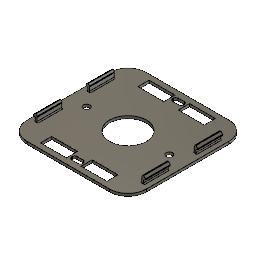
LightSwitch (Autodesk Fusion 360 design; units mm, degrees)
Autodesk Fusion 360 part; units mm, degrees
sketch "Sketch1" plane through (0, 0, 0) normal (0, 1, 0) x (1, 0, 0)
  line L0 (32.5, 32.5) -> (-32.5, -32.5) construction
  line L1 (-32.5, 32.5) -> (32.5, -32.5) construction
  line L2 (25.4289, -32.5) -> (32.5, -25.4289)
  line L3 (32.5, 25.4289) -> (25.4289, 32.5)
  line L4 (-25.4289, 32.5) -> (-32.5, 25.4289)
  line L5 (-32.5, -25.4289) -> (-25.4289, -32.5)
  line L6 (-32.5, 32.5) -> (-32.5, 25.4289)
  line L7 (-32.5, -25.4289) -> (-32.5, -32.5)
  line L8 (-32.5, 25.4289) -> (-32.5, -25.4289)
  line L9 (32.5, 32.5) -> (25.4289, 32.5)
  line L10 (-25.4289, 32.5) -> (-32.5, 32.5)
  line L11 (25.4289, 32.5) -> (-25.4289, 32.5)
  line L12 (-32.5, -32.5) -> (-25.4289, -32.5)
  line L13 (25.4289, -32.5) -> (32.5, -32.5)
  line L14 (-25.4289, -32.5) -> (25.4289, -32.5)
  line L15 (32.5, -32.5) -> (32.5, -25.4289)
  line L16 (32.5, 25.4289) -> (32.5, 32.5)
  line L17 (32.5, -25.4289) -> (32.5, 25.4289)
  line L18 (24.7919, 30.962) -> (-24.7919, 30.962)
  line L19 (-24.7919, 30.962) -> (-30.962, 24.7919)
  line L20 (-30.962, 24.7919) -> (-30.962, -24.7919)
  line L21 (-30.962, -24.7919) -> (-24.7919, -30.962)
  line L22 (-24.7919, -30.962) -> (24.7919, -30.962)
  line L23 (24.7919, -30.962) -> (30.962, -24.7919)
  line L24 (30.962, -24.7919) -> (30.962, 24.7919)
  line L25 (30.962, 24.7919) -> (24.7919, 30.962)
  dimension "d1" = 65
  dimension "d2" = 65
  dimension "d3" = 10
  dimension "d6" = 360
  dimension "d10" = 7.0711
  dimension "d11" = 1.538
extrude "Extrude1" add sketch "Sketch1" along normal blind 1.5 contours L2 L3 L4 L5 L8 L11 L14 L17 | L2 L13 L15 | L5 L7 L12 | L3 L9 L16 | L4 L6 L10 | L18 L19 L20 L21 L22 L23 L24 L25 makes body 1
extrude "Extrude2" add 1 faces at (8.4763, 1.5, 10.8333) along direction (0, 1, 0) blind 10 on bodies 1 bodies 1
delete_face "DeleteFace1" 1 faces at (-32.5, 3.8333, 27.786) on bodies 1
delete_face "DeleteFace2" 1 faces at (27.786, 7.6667, 32.5) on bodies 1
delete_face "DeleteFace3" 1 faces at (32.5, 3.8333, -27.786) on bodies 1
delete_face "DeleteFace4" 1 faces at (-27.786, 3.8333, -32.5) on bodies 1
fillet "Fillet1" radius 5 4 edges at (0, 11.5, 32.5) (-32.5, 11.5, 0) (0, 11.5, -32.5) (32.5, 11.5, 0) on bodies 1
fillet "Fillet1" radius 10 4 edges at (-32.5, 5.75, -32.5) (-32.5, 5.75, 32.5) (32.5, 5.75, 32.5) (32.5, 5.75, -32.5) on bodies 1
shell "Shell1" thickness 1.5 removed faces 0 bodies 1
ref_plane "WorkPlane1" through (28.9645, 1.5, -28.9645) normal (0, 1, 0) x (1, 0, 0)
split "Split1" by plane through (28.9645, 1.5, -28.9645) normal (0, 1, 0) bodies 1 makes body 2 at (9.1667, 11.5, 10.8333)
sketch "Sketch3" plane through (0, 0, 0) normal (0, 0, 1) x (1, 0, 0)
  line L0 (31, 1.5) -> (31, 6.5)
  line L1 (32.5, 6.5) -> (25.4289, 6.5)
  line L2 (31, 1.5) -> (31, 3.5)
  line L3 (31, 3.5) -> (30, 3)
  line L4 (32.5, 1.5) -> (25.4289, 1.5)
  line L5 (31, 1.5) -> (29.9, 1.5)
  line L6 (29.4, 2) -> (29.4, 3.4501)
  line L7 (29.4, 3.4501) -> (29.4, 4)
  line L8 (29.4, 4) -> (30.5, 4)
  line L9 (30.5, 4) -> (29.4, 3.4501)
  line L10 (30, 2.5) -> (30, 3)
  line L11 (31, 1.5) -> (28.5, 1.5)
  line L12 (28.5, 4) -> (28.5, 2)
  arc A0 (29.4, 2) -> (29.9, 1.5) centre (29.9, 2) ccw
  line L13 (28, 1.5) -> (26.4, 1.5)
  arc A1 (28, 1.5) -> (28.5, 2) centre (28, 2) ccw
  line L14 (30, 2.5) -> (31, 1.7)
  line L15 (30.5, 4) -> (30.5, 4.5)
  line L16 (30.5, 4.5) -> (29.5, 5.5)
  line L17 (29.5, 5.5) -> (29, 5.5)
  line L18 (29, 5.5) -> (28.5, 4.5)
  line L19 (28.5, 4.5) -> (28.5, 4)
  dimension "d20" = 0.5
  dimension "d21" = 0.5
  measures "d20" radius of A0
  measures "d21" radius of A1
extrude "Extrude3" add sketch "Sketch3" along normal mid plane 42 contours L4 L6 L7 L8 L11 L12 A0 A1 L15 L16 L17 L18 L19 | L7 L8 L9 bodies 1
extrude "Extrude4" add sketch "Sketch3" along normal mid plane 42 contours L0 L2 L3 L10 L14 bodies 2
extrude "Extrude6" cut sketch "Sketch3" along normal mid plane 15 bodies 2 1
pattern_circular "C-Pattern1" count 2 over 360 about axis through (0, 1.75, 0) along (0, 1, 0) of "Extrude3", "Extrude4", "Extrude6"
sketch "Tornillos" plane through (0, 0, 0) normal (0, 1, 0) x (1, 0, 0)
  line L0 (25.4289, 32.5) -> (-25.4289, 32.5)
  line L1 (-7.6716, 32.5) -> (8, 32.5)
  line L2 (0, 32.5) -> (0, 27.5)
  line L3 (1.75, 29) -> (-1.75, 29)
  line L4 (-3, 27.75) -> (-3, 27.25)
  line L5 (-1.75, 26) -> (1.75, 26)
  line L6 (3, 27.25) -> (3, 27.75)
  line L7 (10.5467, 32.7733) -> (-3, 26) construction
  line L8 (-3, 29) -> (3, 26) construction
  arc A0 (3, 27.75) -> (1.75, 29) centre (1.75, 27.75) ccw
  arc A1 (1.75, 26) -> (3, 27.25) centre (1.75, 27.25) ccw
  arc A2 (-3, 27.25) -> (-1.75, 26) centre (-1.75, 27.25) ccw
  arc A3 (-1.75, 29) -> (-3, 27.75) centre (-1.75, 27.75) ccw
  line L9 (0, 0) -> (9, 0)
  line L10 (-1.75, -26) -> (1.75, -26)
  arc A4 (-3, -27.75) -> (-1.75, -29) centre (-1.75, -27.75) ccw
  line L11 (-3, -27.75) -> (-3, -27.25)
  arc A5 (-1.75, -26) -> (-3, -27.25) centre (-1.75, -27.25) ccw
  line L12 (0, -32.5) -> (0, -27.5)
  line L13 (1.75, -29) -> (-1.75, -29)
  line L14 (3, -27.25) -> (3, -27.75)
  line L15 (-3, -29) -> (3, -26) construction
  arc A6 (1.75, -29) -> (3, -27.75) centre (1.75, -27.75) ccw
  arc A7 (3, -27.25) -> (1.75, -26) centre (1.75, -27.25) ccw
  line L16 (10.5467, -32.7733) -> (-3, -26) construction
  line L17 (32.5, -25.4289) -> (32.5, 25.4289)
  line L18 (32.5, -22.5) -> (32.5, 22.5)
  line L19 (32.5, 0) -> (25.4289, 0)
  line L20 (32.5, -7.15) -> (32.5, 7)
  line L21 (32.5, 0) -> (22.5, 0)
  circle A8 centre (22.5, 0) radius 1.75
  line L22 (0, 0) -> (0, 8)
  circle A9 centre (-22.5, 0) radius 1.75
  dimension "d33" = 6
  dimension "d34" = 3
  dimension "d35" = 1.25
  dimension "d36" = 5
  dimension "d37" = 3
  dimension "d38" = 10
  dimension "d39" = 3.5
  dimension "d43" = 4
  dimension "d44" = 10
  dimension "d45" = 3
  dimension "d46" = 3
  measures "d35" radius of A0
  measures "d37" distance of L3 L5
  measures "d39" diameter of A8
  measures "d44" distance of L11 L14
  measures "d45" distance of L10 L13
  measures "d46" distance of L14
extrude "Extrude7" cut sketch "Tornillos" along normal blind 10 bodies 1
sketch "Encajar" plane through (0, 1.5, 0) normal (0, 1, 0) x (-1, 0, 0)
  line L0 (1.75, -29) -> (-1.75, -29)
  arc A0 (-3, -27.75) -> (-1.75, -29) centre (-1.75, -27.75) ccw
  line L1 (-3, -27.75) -> (-3, -27.25)
  arc A1 (-1.75, -26) -> (-3, -27.25) centre (-1.75, -27.25) ccw
  line L2 (-1.75, -26) -> (1.75, -26)
  arc A2 (3, -27.25) -> (1.75, -26) centre (1.75, -27.25) ccw
  line L3 (3, -27.25) -> (3, -27.75)
  arc A3 (1.75, -29) -> (3, -27.75) centre (1.75, -27.75) ccw
  circle A4 centre (22.5, 0) radius 1.75
  circle A5 centre (-22.5, 0) radius 1.75
  line L4 (-1.75, 29) -> (1.75, 29)
  arc A6 (3, 27.75) -> (1.75, 29) centre (1.75, 27.75) ccw
  line L5 (3, 27.75) -> (3, 27.25)
  arc A7 (1.75, 26) -> (3, 27.25) centre (1.75, 27.25) ccw
  line L6 (1.75, 26) -> (-1.75, 26)
  arc A8 (-3, 27.25) -> (-1.75, 26) centre (-1.75, 27.25) ccw
  line L7 (-3, 27.25) -> (-3, 27.75)
  arc A9 (-1.75, 29) -> (-3, 27.75) centre (-1.75, 27.75) ccw
  line L8 (29.9, -7.5) -> (29.9, -21)
  line L9 (29.9, -21) -> (28, -21)
  line L10 (28, -21) -> (28, -7.5)
  line L11 (28, -7.5) -> (29.9, -7.5)
  line L12 (29.9, 7.5) -> (28, 7.5)
  line L13 (28, 7.5) -> (28, 21)
  line L14 (28, 21) -> (29.9, 21)
  line L15 (29.9, 21) -> (29.9, 7.5)
  line L16 (-29.9, 7.5) -> (-29.9, 21)
  line L17 (-29.9, 21) -> (-28, 21)
  line L18 (-28, 21) -> (-28, 7.5)
  line L19 (-28, 7.5) -> (-29.9, 7.5)
  line L20 (-29.9, -7.5) -> (-28, -7.5)
  line L21 (-28, -7.5) -> (-28, -21)
  line L22 (-28, -21) -> (-29.9, -21)
  line L23 (-29.9, -21) -> (-29.9, -7.5)
  arc A10 (32.5, 22.5) -> (22.5, 32.5) centre (22.5, 22.5) ccw
  line L24 (22.5, 32.5) -> (-22.5, 32.5)
  arc A11 (-22.5, 32.5) -> (-32.5, 22.5) centre (-22.5, 22.5) ccw
  line L25 (-32.5, 22.5) -> (-32.5, -22.5)
  arc A12 (-32.5, -22.5) -> (-22.5, -32.5) centre (-22.5, -22.5) ccw
  line L26 (-22.5, -32.5) -> (22.5, -32.5)
  arc A13 (22.5, -32.5) -> (32.5, -22.5) centre (22.5, -22.5) ccw
  line L27 (32.5, -22.5) -> (32.5, 22.5)
  line L28 (-32.5, 32.5) -> (32.5, 32.5)
  line L29 (32.5, 32.5) -> (32.5, -32.5)
  line L30 (32.5, -32.5) -> (-32.5, -32.5)
  line L31 (-32.5, -32.5) -> (-32.5, 32.5)
  line L32 (-32.5, 32.5) -> (32.5, -32.5) construction
  line L33 (32.5, 32.5) -> (-32.5, -32.5) construction
  line L34 (18, -29.5) -> (4, -29.5)
  line L35 (4, -29.5) -> (4, -23.5)
  line L36 (4, -23.5) -> (18, -23.5)
  line L37 (18, -23.5) -> (18, -29.5)
  line L38 (0, 0) -> (-9, 0)
  line L39 (0, 0) -> (0, -5)
  line L40 (0, 0) -> (-4.5, 0)
  line L41 (-4, -23.5) -> (-18, -23.5)
  line L42 (-4, -29.5) -> (-4, -23.5)
  line L43 (-18, -29.5) -> (-4, -29.5)
  line L44 (-18, -23.5) -> (-18, -29.5)
  line L45 (-4, 23.5) -> (-18, 23.5)
  line L46 (-4, 29.5) -> (-4, 23.5)
  line L47 (-18, 29.5) -> (-4, 29.5)
  line L48 (-18, 23.5) -> (-18, 29.5)
  line L49 (4, 23.5) -> (18, 23.5)
  line L50 (4, 29.5) -> (4, 23.5)
  line L51 (18, 29.5) -> (4, 29.5)
  line L52 (18, 23.5) -> (18, 29.5)
  dimension "d47" = 65
  dimension "d48" = 65
  dimension "d49" = 14
  dimension "d50" = 6
  dimension "d51" = 14.5
  dimension "d52" = 3
  dimension "d54" = 360
  measures "d51" distance of L29 L37
  measures "d52" distance of L30 L34
extrude "Extrude8" cut sketch "Encajar" against normal blind 10 contours L34 L35 L36 L37 | L41 L42 L43 L44 | L45 L46 L47 L48 | L49 L50 L51 L52 bodies 1
sketch "Agujeros" plane through (0, 1.5, 0) normal (0, 1, 0) x (-1, 0, 0)
  line L0 (-4, -29.5) -> (-18, -29.5)
  line L1 (-18, -29.5) -> (-18, -23.5)
  line L2 (-18, -23.5) -> (-4, -23.5)
  line L3 (-4, -23.5) -> (-4, -29.5)
  line L4 (4, 29.5) -> (18, 29.5)
  line L5 (18, 29.5) -> (18, 23.5)
  line L6 (18, 23.5) -> (4, 23.5)
  line L7 (4, 23.5) -> (4, 29.5)
  line L8 (4, -29.5) -> (4, -23.5)
  line L9 (4, -23.5) -> (18, -23.5)
  line L10 (18, -23.5) -> (18, -29.5)
  line L11 (18, -29.5) -> (4, -29.5)
  line L12 (-4, 29.5) -> (-4, 23.5)
  line L13 (-4, 23.5) -> (-18, 23.5)
  line L14 (-18, 23.5) -> (-18, 29.5)
  line L15 (-18, 29.5) -> (-4, 29.5)
  line L16 (1.75, -29) -> (-1.75, -29)
  arc A0 (-3, -27.75) -> (-1.75, -29) centre (-1.75, -27.75) ccw
  line L17 (-3, -27.75) -> (-3, -27.25)
  arc A1 (-1.75, -26) -> (-3, -27.25) centre (-1.75, -27.25) ccw
  line L18 (-1.75, -26) -> (1.75, -26)
  arc A2 (3, -27.25) -> (1.75, -26) centre (1.75, -27.25) ccw
  line L19 (3, -27.25) -> (3, -27.75)
  arc A3 (1.75, -29) -> (3, -27.75) centre (1.75, -27.75) ccw
  circle A4 centre (22.5, 0) radius 1.75
  circle A5 centre (-22.5, 0) radius 1.75
  line L20 (-1.75, 29) -> (1.75, 29)
  arc A6 (3, 27.75) -> (1.75, 29) centre (1.75, 27.75) ccw
  line L21 (3, 27.75) -> (3, 27.25)
  arc A7 (1.75, 26) -> (3, 27.25) centre (1.75, 27.25) ccw
  line L22 (1.75, 26) -> (-1.75, 26)
  arc A8 (-3, 27.25) -> (-1.75, 26) centre (-1.75, 27.25) ccw
  line L23 (-3, 27.25) -> (-3, 27.75)
  arc A9 (-1.75, 29) -> (-3, 27.75) centre (-1.75, 27.75) ccw
  line L24 (29.9, -7.5) -> (29.9, -21)
  line L25 (29.9, -21) -> (28, -21)
  line L26 (28, -21) -> (28, -7.5)
  line L27 (28, -7.5) -> (29.9, -7.5)
  line L28 (29.9, 7.5) -> (28, 7.5)
  line L29 (28, 7.5) -> (28, 21)
  line L30 (28, 21) -> (29.9, 21)
  line L31 (29.9, 21) -> (29.9, 7.5)
  line L32 (-29.9, 7.5) -> (-29.9, 21)
  line L33 (-29.9, 21) -> (-28, 21)
  line L34 (-28, 21) -> (-28, 7.5)
  line L35 (-28, 7.5) -> (-29.9, 7.5)
  line L36 (-29.9, -7.5) -> (-28, -7.5)
  line L37 (-28, -7.5) -> (-28, -21)
  line L38 (-28, -21) -> (-29.9, -21)
  line L39 (-29.9, -21) -> (-29.9, -7.5)
  arc A10 (32.5, 22.5) -> (22.5, 32.5) centre (22.5, 22.5) ccw
  line L40 (22.5, 32.5) -> (-22.5, 32.5)
  arc A11 (-22.5, 32.5) -> (-32.5, 22.5) centre (-22.5, 22.5) ccw
  line L41 (-32.5, 22.5) -> (-32.5, -22.5)
  arc A12 (-32.5, -22.5) -> (-22.5, -32.5) centre (-22.5, -22.5) ccw
  line L42 (-22.5, -32.5) -> (22.5, -32.5)
  arc A13 (22.5, -32.5) -> (32.5, -22.5) centre (22.5, -22.5) ccw
  line L43 (32.5, -22.5) -> (32.5, 22.5)
  circle A14 centre (0, 0) radius 10
  dimension "d57" = 20
  measures "d57" diameter of A14
extrude "Extrude9" cut sketch "Agujeros" against normal blind 5 contours A14 bodies 1
sketch "Sketch9" plane through (0, 0, -32.5) normal (0, 0, -1) x (-1, 0, 0)
  line L0 (-22.5, 1.5) -> (22.5, 1.5)
  line L1 (22.5, 1.5) -> (22.5, 6.5)
  line L2 (22.5, 6.5) -> (-22.5, 6.5)
  line L3 (-22.5, 6.5) -> (-22.5, 1.5)
  line L4 (9.5, 6) -> (17.5, 6)
  line L5 (17.5, 6) -> (17.5, 10)
  line L6 (17.5, 10) -> (9.5, 10)
  line L7 (9.5, 10) -> (9.5, 6)
  line L8 (-22.5, 0) -> (22.5, 0)
  line L9 (32.5, 1.5) -> (32.5, 6.5)
  dimension "d64" = 8
  dimension "d65" = 4
  dimension "d66" = 6
  dimension "d67" = 15
  measures "d66" distance of L4 L8
  measures "d67" distance of L5 L9
extrude "Extrude10" cut sketch "Sketch9" against normal blind 9 contours L2 L5 L6 L7 bodies 2
hidden bodies 2
equation "d1 = d2"
equation "d46 = d33 / 2"
